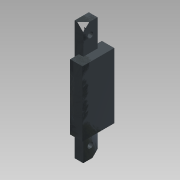
# Autodesk Inventor part: 90_Linearführung
Saved by Autodesk Inventor 2015 (Build 190159000, 159)
## iProperties
Created: 2016-03-16
Part Number: 90_Linearführung
Material: Eisen, grau
Document SubType Name: Modeling
Designer: Bene
Density: 7.15 g/cm^3
Appearance: Eisen - grau
Author: Bene
Autodesk Inventor part; units mm, degrees
ref_plane "YZ Plane" through (0, 0, 0) normal (1, 0, 0) x (0, 1, 0)
ref_plane "XZ Plane" through (0, 0, 0) normal (0, 1, 0) x (-1, 0, 0)
ref_plane "XY Plane" through (0, 0, 0) normal (0, 0, 1) x (1, 0, 0)
sketch "Skizze1" plane through (0, 0, 0) normal (1, 0, 0) x (0, 1, 0)
  line L0 (0, 0) -> (9, 0)
  line L1 (9, 0) -> (9, 75)
  line L2 (9, 75) -> (0, 75)
  line L3 (0, 75) -> (0, 0)
  dimension "d0" = 9
  dimension "d1" = 75
  constraints: 8 end point, 2 parallel, 1 horizontal, 1 perpendicular
  measures "d0" distance of L2.end L1.end
  measures "d1" distance of L1.end L0.end
extrude "Extrusion1" add sketch "Skizze1" along normal blind 5.5
sketch "Skizze2" plane through (5.5, 0, 0) normal (1, 0, 0) x (0, 0, -1)
  line L0 (0, 0) -> (0, 9) projected
  line L1 (0, 9) -> (-75, 9) projected
  line L2 (-75, 9) -> (-75, 0) projected
  line L3 (-75, 0) -> (0, 0) projected
  circle A0 centre (-67.5, 4.5) radius 1.75
  circle A1 centre (-7.5, 4.5) radius 1.75
  circle A2 centre (-47.5, 4.5) radius 1.75
  circle A3 centre (-27.5, 4.5) radius 1.75
  dimension "d4" = 3.5
  dimension "d5" = 7.5
  dimension "d6" = 3.5
  dimension "d7" = 7.5
  dimension "d8" = 3.5
  dimension "d9" = 20
  dimension "d10" = 3.5
  dimension "d11" = 20
  constraints: 4 centre point
  measures "d4" diameter of A0
  measures "d5" distance from line of L2 A0.centre
  measures "d6" diameter of A1
  measures "d7" distance from line of A1.centre L0
  measures "d8" diameter of A2
  measures "d9" distance of A2.centre A0.centre
  measures "d10" diameter of A3
  measures "d11" distance of A3.centre A1.centre
extrude "Extrusion2" cut sketch "Skizze2" against normal through all contours A0 | A1 | A2 | A3
sketch "Skizze3" plane through (5.5, 0, 0) normal (1, 0, 0) x (0, 0, -1)
  circle A0 centre (-47.5, 4.5) radius 1.75 projected
  circle A1 centre (-67.5, 4.5) radius 1.75 projected
  circle A2 centre (-7.5, 4.5) radius 1.75 projected
  circle A3 centre (-27.5, 4.5) radius 1.75 projected
  line L0 (0, 0) -> (0, 9) projected
  line L1 (0, 9) -> (-75, 9) projected
  line L2 (-75, 9) -> (-75, 0) projected
  line L3 (-75, 0) -> (0, 0) projected
  line L4 (-58, 14.5) -> (-17, 14.5)
  line L5 (-17, 14.5) -> (-17, -5.5)
  line L6 (-17, -5.5) -> (-58, -5.5)
  line L7 (-58, -5.5) -> (-58, 14.5)
  line L8 (-58, 14.5) -> (-17, -5.5) construction
  line L9 (-17, 14.5) -> (-58, -5.5) construction
  point P0 (-37.5, 4.5)
  dimension "d15" = 41
  dimension "d16" = 20
  constraints: 12 end point, 2 midpoint, 2 parallel, 1 horizontal, 1 perpendicular
  measures "d15" distance of L5.end L6.end
  measures "d16" distance of L4.end L5.end
extrude "Extrusion3" add sketch "Skizze3" along normal blind 5 and the other way blind 2.75 contours A0 | A3 | L5 L6 L7 L3 | L3 L7 L1 L5 | L1 L7 L4 L5
